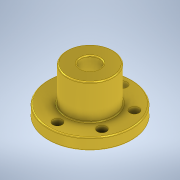
# Autodesk Inventor part: Trapezmutter_T8_ganz
Saved by Autodesk Inventor 2022 (Build 260153000, 153)
## iProperties
Created: 2021-04-21
Part Number: Trapezmutter_T8_ganz
Material: Generic
Document SubType Name: Modeling
Designer: Fabijan_Sven
Density: 1 g/cm^3
Appearance: Metal 2400F Hot
Author: Fabijan_Sven
Autodesk Inventor part; units mm, degrees
ref_plane "YZ Plane" through (0, 0, 0) normal (1, 0, 0) x (0, 1, 0)
ref_plane "XZ Plane" through (0, 0, 0) normal (0, 1, 0) x (-1, 0, 0)
ref_plane "XY Plane" through (0, 0, 0) normal (0, 0, 1) x (1, 0, 0)
sketch "Sketch1" plane through (0, 0, 0) normal (0, 1, 0) x (-1, 0, 0)
  circle A0 centre (0, 0) radius 18
  dimension "d0" = 36
  constraints: 1 centre point, 1 coincident
  measures "d0" diameter of A0
extrude "Extrusion1" add sketch "Sketch1" along normal blind 5
sketch "Sketch2" plane through (0, 5, 0) normal (0, 1, 0) x (1, 0, 0)
  circle A0 centre (0, 0) radius 10
  dimension "d3" = 20
  constraints: 1 centre point, 1 coincident
  measures "d3" diameter of A0
extrude "Extrusion2" add sketch "Sketch2" along normal blind 15
sketch "Sketch3" plane through (0, 20, 0) normal (0, 1, 0) x (1, 0, 0)
  point P0 (0, 0)
hole "Hole1" at (0, 20, 0) direction (0, -1, 0) diameter 8 end through all
sketch "Sketch4" plane through (0, 5, 0) normal (0, 1, 0) x (1, 0, 0)
  circle A0 centre (0, 0) radius 14
  circle A1 centre (0, -14) radius 2
  circle A2 centre (12.1244, -7) radius 2
  circle A3 centre (12.1244, 7) radius 2
  circle A4 centre (0, 14) radius 2
  circle A5 centre (-12.1244, 7) radius 2
  circle A6 centre (-12.1244, -7) radius 2
  dimension "d13" = 28
  dimension "d14" = 4
  dimension "d17" = 360
  constraints: 6 centre point, 1 coincident, 1 vertical alignment, 15 other
  measures "d14" diameter of A1
hole "Hole2" at (0, 5, -14) at (0, 5, 14) at (12.1244, 5, 7) at (12.1244, 5, -7) direction (0, -1, 0) diameter 4 end through all
fillet "Fillet1" radius 0.5 6 edges at (0, 20, -4) (-10, 20, 0) (-10, 5, 0) (18, 5, 0) (18, 0, 0) (0, 0, -4)
equation "\"d19\" = d14"
body "Solid1"
